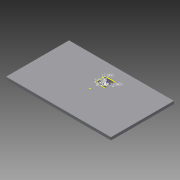
# Autodesk Inventor part: East_Structure_Roof_Devices
Saved by Autodesk Inventor 2013 SP2 (Build 170200200, 200)
## iProperties
Created: 2014-07-16
Part Number: East_Structure_Roof_Devices
Material: Generic
Document SubType Name: Modeling
Designer: jmw3
Density: 1 g/cm^3
Author: jmw3
Autodesk Inventor part; units mm, degrees
ref_plane "YZ Plane" through (0, 0, 0) normal (1, 0, 0) x (0, 1, 0)
ref_plane "XZ Plane" through (0, 0, 0) normal (0, 1, 0) x (-1, 0, 0)
ref_plane "XY Plane" through (0, 0, 0) normal (0, 0, 1) x (1, 0, 0)
sketch "Sketch1" plane through (0, 0, 0) normal (0, 1, 0) x (-1, 0, 0)
  line L0 (3657.6, -6096) -> (3657.6, 6096)
  line L1 (-3657.6, 6096) -> (-3657.6, -6096)
  line L2 (-3657.6, -6096) -> (-609.6, -6096)
  line L3 (609.6, -6096) -> (3657.6, -6096)
  line L4 (3657.6, 6096) -> (914.4, 6096)
  line L5 (-914.4, 6096) -> (-3657.6, 6096)
  line L6 (0, -8534.4) -> (0, 8534.4) projected
  line L7 (-5120.64, 0) -> (5120.64, 0) projected
  line L8 (-3657.6, -6096) -> (3657.6, -6096)
  line L9 (3657.6, -6096) -> (3657.6, 6096)
  line L10 (3657.6, 6096) -> (-3657.6, 6096)
  line L11 (-3657.6, 6096) -> (-3657.6, -6096)
  line L12 (-2133.6, -406.4) -> (-965.2, -406.4)
  line L13 (-965.2, -406.4) -> (-965.2, 762)
  line L14 (-965.2, 762) -> (-2133.6, 762)
  line L15 (-2133.6, 762) -> (-2133.6, -406.4)
  dimension "d0" = 7315.2
  dimension "d12" = 12192
  dimension "d16" = 1168.4
  dimension "d17" = 1168.4
  dimension "d18" = 1524
  dimension "d19" = 5689.6
  constraints: 28 end point, 9 parallel, 4 horizontal, 4 perpendicular, 2 collinear, 2 other
  measures "d0" distance between parallel lines of L0 L1
  measures "d12" distance between parallel lines of L3 L4
  measures "d16" distance between parallel lines of L14 L12
  measures "d17" distance between parallel lines of L13 L15
  measures "d18" distance between parallel lines of L1 L15
  measures "d19" distance between parallel lines of L2 L12
extrude "Extrusion1" add sketch "Sketch1" along normal blind 304.8 contours L3 L8 L6 L7 L0 | L7 L6 L10 L4 L0 | L7 L13 L14 L15 L1 L5 L10 L6 | L6 L8 L2 L1 L7 L15 L12 L13
sketch "Sketch2" plane through (0, 0, 0) normal (0, -1, 0) x (1, 0, 0)
  line L0 (3657.6, -6096) -> (3657.6, 6096)
  line L1 (-3657.6, 6096) -> (-3657.6, -6096)
  line L2 (-3048, 1714.5) -> (-3048, -1714.5)
  line L3 (3048, -5486.4) -> (3048, -1828.8)
  line L4 (3048, -1714.5) -> (3048, 1714.5)
  line L5 (3048, 1828.8) -> (3048, 5486.4)
  line L6 (-3048, -1828.8) -> (-3048, -5486.4)
  line L7 (-3048, 5486.4) -> (-3048, 1828.8)
  line L8 (-3048, 1714.5) -> (-3048, -1714.5)
  line L9 (-2009.775, -1828.8) -> (-2009.775, -1714.5)
  line L10 (-1095.375, -1828.8) -> (-1095.375, -1714.5)
  line L11 (-3048, -1714.5) -> (-2009.775, -1714.5)
  line L12 (-1095.375, -1714.5) -> (-57.15, -1714.5)
  line L13 (-3048, -1828.8) -> (-2009.775, -1828.8)
  line L14 (3048, -1714.5) -> (2009.775, -1714.5)
  line L15 (3048, -1828.8) -> (2009.775, -1828.8)
  line L16 (2009.775, -1828.8) -> (2009.775, -1714.5)
  line L17 (1095.375, -1828.8) -> (1095.375, -1714.5)
  line L18 (1095.375, -1714.5) -> (57.15, -1714.5)
  line L19 (1095.375, -1828.8) -> (-1095.375, -1828.8)
  line L20 (-2009.775, -1828.8) -> (-3048, -1828.8)
  line L21 (-1095.375, -1828.8) -> (1095.375, -1828.8)
  line L22 (2009.775, -1828.8) -> (3048, -1828.8)
  line L23 (57.15, -1714.5) -> (1095.375, -1714.5)
  line L24 (2009.775, -1714.5) -> (3048, -1714.5)
  line L25 (2009.775, 1828.8) -> (3048, 1828.8)
  line L26 (3048, 1828.8) -> (2009.775, 1828.8)
  line L27 (3048, 1714.5) -> (2009.775, 1714.5)
  line L28 (2009.775, 1714.5) -> (3048, 1714.5)
  line L29 (1095.375, 1714.5) -> (57.15, 1714.5)
  line L30 (-1095.375, 1828.8) -> (-1095.375, 1714.5)
  line L31 (-3048, 1714.5) -> (-2009.775, 1714.5)
  line L32 (-1095.375, 1714.5) -> (-57.15, 1714.5)
  line L33 (-3048, 1828.8) -> (-2009.775, 1828.8)
  line L34 (2009.775, 1828.8) -> (2009.775, 1714.5)
  line L35 (1095.375, 1828.8) -> (1095.375, 1714.5)
  line L36 (1095.375, 1828.8) -> (-1095.375, 1828.8)
  line L37 (-2009.775, 1828.8) -> (-3048, 1828.8)
  line L38 (-1095.375, 1828.8) -> (1095.375, 1828.8)
  line L39 (57.15, 1714.5) -> (1095.375, 1714.5)
  line L40 (-2009.775, 1828.8) -> (-2009.775, 1714.5)
  line L41 (-57.15, -457.2) -> (57.15, -457.2)
  line L42 (57.15, 457.2) -> (-57.15, 457.2)
  line L43 (-609.6, -6096) -> (-609.6, -5486.4)
  line L44 (609.6, -6096) -> (609.6, -5486.4)
  line L45 (-3048, -5486.4) -> (-609.6, -5486.4)
  line L46 (609.6, -5486.4) -> (3048, -5486.4)
  line L47 (-3657.6, -6096) -> (-609.6, -6096)
  line L48 (609.6, -6096) -> (3657.6, -6096)
  line L49 (914.4, 5486.4) -> (914.4, 6096)
  line L50 (-914.4, 6096) -> (-914.4, 5486.4)
  line L51 (3048, 5486.4) -> (914.4, 5486.4)
  line L52 (-914.4, 5486.4) -> (-3048, 5486.4)
  line L53 (3657.6, 6096) -> (914.4, 6096)
  line L54 (-914.4, 6096) -> (-3657.6, 6096)
  line L55 (-57.15, -1714.5) -> (-57.15, -457.2)
  line L56 (-57.15, 457.2) -> (-57.15, 1714.5)
  line L57 (-57.15, 1714.5) -> (-57.15, 457.2)
  line L58 (-57.15, -457.2) -> (-57.15, -1714.5)
  line L59 (57.15, -1714.5) -> (57.15, -457.2)
  line L60 (57.15, 457.2) -> (57.15, 1714.5)
  line L61 (57.15, 1714.5) -> (57.15, 457.2)
  line L62 (57.15, -457.2) -> (57.15, -1714.5)
  line L63 (-3048, 5486.4) -> (-3048, 1828.8)
  line L64 (-3048, 1828.8) -> (-2009.775, 1828.8)
  line L65 (-2009.775, 1828.8) -> (-2009.775, 1714.5)
  line L66 (-2009.775, 1714.5) -> (-3048, 1714.5)
  line L67 (-3048, 1714.5) -> (-3048, -1714.5)
  line L68 (-3048, -1714.5) -> (-2009.775, -1714.5)
  line L69 (-2009.775, -1714.5) -> (-2009.775, -1828.8)
  line L70 (-2009.775, -1828.8) -> (-3048, -1828.8)
  line L71 (-3048, -1828.8) -> (-3048, -5486.4)
  line L72 (-3048, -5486.4) -> (-609.6, -5486.4)
  line L73 (609.6, -5486.4) -> (3048, -5486.4)
  line L74 (3048, -5486.4) -> (3048, -1828.8)
  line L75 (3048, -1828.8) -> (2009.775, -1828.8)
  line L76 (2009.775, -1828.8) -> (2009.775, -1714.5)
  line L77 (2009.775, -1714.5) -> (3048, -1714.5)
  line L78 (3048, 1714.5) -> (3048, -1714.5)
  line L79 (3048, 1714.5) -> (2009.775, 1714.5)
  line L80 (2009.775, 1714.5) -> (2009.775, 1828.8)
  line L81 (2009.775, 1828.8) -> (3048, 1828.8)
  line L82 (3048, 1828.8) -> (3048, 5486.4)
  line L83 (3657.6, 6096) -> (-3657.6, 6096) projected
  line L84 (0, 8534.4) -> (0, -8534.4) projected
  line L85 (-12.7, 6096) -> (12.7, 6096)
  line L86 (3657.6, -6096) -> (3657.6, 6096) projected
  line L87 (-2009.775, 1828.8) -> (-2008.505, 1828.8)
  line L88 (-1095.375, 1828.8) -> (-1096.645, 1828.8)
  line L89 (-1095.375, 1714.5) -> (-1096.645, 1714.5)
  line L90 (-1096.645, 1714.5) -> (-1096.645, 1828.8)
  line L91 (-2009.775, 1714.5) -> (-2008.505, 1714.5)
  line L92 (-2008.505, 1714.5) -> (-2008.505, 1828.8)
  line L93 (-2008.505, 1828.8) -> (-1096.645, 1828.8)
  line L94 (-1096.645, 1828.8) -> (-1096.645, 1714.5)
  line L95 (-1096.645, 1714.5) -> (-2008.505, 1714.5)
  line L96 (-2008.505, 1714.5) -> (-2008.505, 1828.8)
  line L97 (-5120.64, 0) -> (5120.64, 0) projected
  line L98 (-2009.775, -1828.8) -> (-2008.505, -1828.8)
  line L99 (-1095.375, -1828.8) -> (-1096.645, -1828.8)
  line L100 (-1095.375, -1714.5) -> (-1096.645, -1714.5)
  line L101 (-2009.775, -1714.5) -> (-2008.505, -1714.5)
  line L102 (-2008.505, -1714.5) -> (-2008.505, -1828.8)
  line L103 (-2008.505, -1828.8) -> (-1096.645, -1828.8)
  line L104 (-1096.645, -1828.8) -> (-1096.645, -1714.5)
  line L105 (-1096.645, -1714.5) -> (-2008.505, -1714.5)
  line L106 (2009.775, 1828.8) -> (2008.505, 1828.8)
  line L107 (1095.375, 1828.8) -> (1096.645, 1828.8)
  line L108 (1095.375, 1714.5) -> (1096.645, 1714.5)
  line L109 (1096.645, 1714.5) -> (1096.645, 1828.8)
  line L110 (2009.775, 1714.5) -> (2008.505, 1714.5)
  line L111 (2008.505, 1714.5) -> (2008.505, 1828.8)
  line L112 (2008.505, 1828.8) -> (1096.645, 1828.8)
  line L113 (1096.645, 1714.5) -> (2008.505, 1714.5)
  line L114 (2009.775, -1714.5) -> (2008.505, -1714.5)
  line L115 (2008.505, -1714.5) -> (2008.505, -1828.8)
  line L116 (2009.775, -1828.8) -> (2008.505, -1828.8)
  line L117 (2008.505, -1828.8) -> (1096.645, -1828.8)
  line L118 (1096.645, -1714.5) -> (2008.505, -1714.5)
  line L119 (1095.375, -1714.5) -> (1096.645, -1714.5)
  line L120 (1096.645, -1828.8) -> (1096.645, -1714.5)
  line L121 (1095.375, -1828.8) -> (1096.645, -1828.8)
  line L122 (-3657.6, 6096) -> (-3657.6, -6096) projected
  line L123 (-3657.6, -6096) -> (3657.6, -6096) projected
  line L124 (-2008.505, -1828.8) -> (-1096.645, -1828.8)
  line L125 (-1096.645, -1828.8) -> (-1096.645, -1714.5)
  line L126 (-1096.645, -1714.5) -> (-2008.505, -1714.5)
  line L127 (-2008.505, -1714.5) -> (-2008.505, -1828.8)
  line L128 (1096.645, -1714.5) -> (2008.505, -1714.5)
  line L129 (2008.505, -1714.5) -> (2008.505, -1828.8)
  line L130 (2008.505, -1828.8) -> (1096.645, -1828.8)
  line L131 (1096.645, -1828.8) -> (1096.645, -1714.5)
  line L132 (1096.645, 1828.8) -> (2008.505, 1828.8)
  line L133 (2008.505, 1828.8) -> (2008.505, 1714.5)
  line L134 (2008.505, 1714.5) -> (1096.645, 1714.5)
  line L135 (1096.645, 1714.5) -> (1096.645, 1828.8)
  line L136 (-912.876, 6096) -> (-12.7, 6096)
  line L137 (-12.7, 6096) -> (-12.7, 5486.4)
  line L138 (-12.7, 5486.4) -> (-912.876, 5486.4)
  line L139 (-912.876, 5486.4) -> (-912.876, 6096)
  line L140 (12.7, 6096) -> (12.7, 5486.4)
  line L141 (12.7, 5486.4) -> (912.876, 5486.4)
  line L142 (912.876, 5486.4) -> (912.876, 6096)
  line L143 (-912.876, 5486.4) -> (-12.7, 5486.4)
  line L144 (-12.7, 5486.4) -> (-12.7, 6096)
  line L145 (-12.7, 6096) -> (-912.876, 6096)
  line L146 (-912.876, 6096) -> (-912.876, 5486.4)
  line L147 (12.7, 6096) -> (912.876, 6096)
  line L148 (912.876, 6096) -> (912.876, 5486.4)
  line L149 (912.876, 5486.4) -> (12.7, 5486.4)
  line L150 (12.7, 5486.4) -> (12.7, 6096)
  line L151 (-608.33, -5486.4) -> (608.33, -5486.4)
  line L152 (608.33, -5486.4) -> (608.33, -6096)
  line L153 (608.33, -6096) -> (-608.33, -6096)
  line L154 (-608.33, -6096) -> (-608.33, -5486.4)
  line L155 (-3657.6, 609.6) -> (-3048, 609.6)
  line L156 (-3048, 609.6) -> (-3048, -609.6)
  line L157 (-3048, -609.6) -> (-3657.6, -609.6)
  line L158 (-3657.6, -609.6) -> (-3657.6, 609.6)
  line L159 (-57.15, 455.93) -> (57.15, 455.93)
  line L160 (57.15, 455.93) -> (57.15, -455.93)
  line L161 (57.15, -455.93) -> (-57.15, -455.93)
  line L162 (-57.15, -455.93) -> (-57.15, 455.93)
  line L163 (-3657.6, 608.33) -> (-3048, 608.33)
  line L164 (-3048, 608.33) -> (-3048, -608.33)
  line L165 (-3048, -608.33) -> (-3657.6, -608.33)
  line L166 (-3657.6, -608.33) -> (-3657.6, 608.33)
  point P0 (0, 0)
  point P1 (0, 0)
  point P2 (0, 5486.4)
  dimension "d22" = 7315.2
  dimension "d23" = 609.6
  dimension "d24" = 1038.225
  dimension "d25" = 914.4
  dimension "d26" = 114.3
  dimension "d27" = 1038.225
  dimension "d28" = 1038.225
  dimension "d29" = 914.4
  dimension "d30" = 1219.2
  dimension "d31" = 609.6
  dimension "d32" = 4267.2
  dimension "d33" = 1828.8
  dimension "d34" = 12192
  dimension "d35" = 609.6
  dimension "d36" = 114.3
  dimension "d40" = 1.27
  dimension "d41" = 1.27
  dimension "d42" = 1.524
  dimension "d43" = 12.7
  dimension "d44" = 1.27
  dimension "d45" = 1219.2
  dimension "d48" = 1.27
  dimension "d51" = 1.27
  constraints: 322 end point, 60 perpendicular, 45 parallel, 24 collinear, 22 symmetric about line, 19 horizontal, 8 point on line, 4 other
  measures "d22" distance between parallel lines of L0 L1
  measures "d23" distance between parallel lines of L0 L3
  measures "d24" distance between parallel lines of L8 L9
  measures "d25" distance between parallel lines of L9 L10
  measures "d26" distance between parallel lines of L21 L18
  measures "d27" distance of L66.end L40.end
  measures "d28" distance of L4.end L27.end
  measures "d29" distance between parallel lines of L41 L42
  measures "d30" distance between parallel lines of L44 L43
  measures "d31" distance between parallel lines of L47 L45
  measures "d32" distance between parallel lines of L13 L47
  measures "d33" distance between parallel lines of L49 L50
  measures "d34" distance between parallel lines of L48 L53
  measures "d35" distance between parallel lines of L54 L52
  measures "d36" distance between parallel lines of L62 L55
  measures "d40" distance of L36.end L88.end
  measures "d41" distance of L40.start L87.end
  measures "d42" distance between parallel lines of L50 L139
  measures "d43" distance between parallel lines of L84 L137
  measures "d44" distance between parallel lines of L43 L154
  measures "d45" distance between parallel lines of L157 L155
  measures "d48" distance between parallel lines of L42 L159
  measures "d51" distance between parallel lines of L155 L163
extrude "Extrusion3" add sketch "Sketch2" along normal blind 19.05 contours L48 L44 L46 L3 L15 L16 L14 L4 L97 L0 | L97 L4 L27 L34 L25 L5 L51 L49 L53 L0 | L123 L84 L151 L152 | L123 L154 L151 L84 | L142 L141 L140 L83 | L115 L117 L120 L118 | L113 L109 L112 L111 | L84 L41 L59 L18 L17 L19 | L19 L10 L12 L55 L41 L84 | L47 L1 L157 L2 L11 L9 L13 L6 L45 L43 | L84 L36 L35 L29 L60 L42 | L42 L56 L32 L30 L36 L84 | L97 L1 L163 L2 | L2 L165 L1 L97 | L137 L138 L139 L83 | L103 L102 L105 L104 | L155 L1 L54 L50 L52 L7 L33 L40 L31 L2 | L90 L95 L92 L93
extrude "Extrusion4" add sketch "Sketch2" along normal blind 19.05 contours L160 L161 L84 L97 | L97 L84 L159 L160 | L97 L162 L159 L84 | L84 L161 L162 L97
sketch "Sketch3" plane through (0, 304.8, 0) normal (0, 1, 0) x (1, 0, 0)
  line L0 (2133.6, 406.4) -> (2133.6, -762) projected
  line L1 (965.2, -762) -> (965.2, 406.4) projected
  line L2 (965.2, 406.4) -> (2133.6, 406.4) projected
  circle A0 centre (1549.4, -177.8) radius 152.4
  line L3 (1333.5, 38.1) -> (1765.3, 38.1)
  line L4 (1333.5, -393.7) -> (1333.5, 38.1)
  line L5 (1765.3, 38.1) -> (1333.5, -393.7)
  point P0 (0, 0)
  dimension "d52" = 304.8
  dimension "d53" = 584.2
  dimension "d54" = 584.2
  dimension "d57" = 368.3
  dimension "d58" = 368.3
  dimension "d59" = 431.8
  constraints: 6 end point, 1 centre point, 1 horizontal, 1 midpoint
  measures "d52" diameter of A0
  measures "d53" distance from line of L2 A0.centre
  measures "d54" distance from line of L0 A0.centre
  measures "d57" distance between parallel lines of L2 L3
  measures "d58" distance between parallel lines of L1 L4
  measures "d59" distance of L4.start L3.start
extrude "Extrusion5" add sketch "Sketch3" along normal blind 76.2 contours A0 L5 | L5 A0
extrude "Extrusion6" add sketch "Sketch3" along normal blind 50.8 contours L5 A0 | A0 L5 L4 L3 picked at (1566.1782, -129.8507)
body "Solid1"
